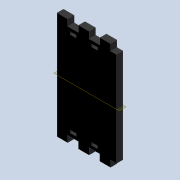
# Autodesk Inventor part: 00_Baseplate_Simmo_side6_v2
Saved by Autodesk Inventor 2022 (Build 260153000, 153)
## iProperties
Created: 2022-08-09
Part Number: 00_Baseplate_Simmo_side6_v2
Material: Generic
Document SubType Name: Modeling
Designer: wanghaoran
Density: 1 g/cm^3
Appearance: Default
Author: wanghaoran
Autodesk Inventor part; units mm, degrees
ref_plane "YZ Plane" through (0, 0, 0) normal (1, 0, 0) x (0, 1, 0)
ref_plane "XZ Plane" through (0, 0, 0) normal (0, 1, 0) x (-1, 0, 0)
ref_plane "XY Plane" through (0, 0, 0) normal (0, 0, 1) x (1, 0, 0)
sketch "Sketch1" plane through (0, 0, 0) normal (0, 0, 1) x (1, 0, 0)
  line L0 (50, 0) -> (55.5309, 0) projected
  line L1 (0, 0) -> (0, 6) projected
  line L2 (0, 0) -> (0, 6) projected
  line L3 (0, 0) -> (0, 6) projected
  line L4 (0, 6) -> (55.5309, 6)
  line L5 (55.5309, 6) -> (55.5309, -94)
  line L6 (55.5309, -94) -> (0, -94)
  line L7 (0, -94) -> (0, 6)
  line L8 (55.5309, 6) -> (55.5309, 0) projected
  line L9 (55.5309, 6) -> (55.5309, 0) projected
  dimension "d16" = 100
  constraints: 8 end point, 2 parallel, 1 horizontal, 1 perpendicular
  measures "d16" distance of L4.end L5.end
extrude "Extrusion1" add sketch "Sketch1" along normal blind 6
sketch "Sketch2" plane through (0, 0, 6) normal (0, 0, 1) x (1, 0, 0)
  line L0 (50, 0) -> (55.5309, 0) projected
  line L1 (50, 6) -> (50, 0) projected
  line L2 (58.2654, -73) -> (58.2654, 6) projected
  line L3 (58.2654, 6) -> (0, 6) projected
  line L4 (30, 6) -> (30, 0) projected
  line L5 (30, 0) -> (40, 0) projected
  line L6 (40, 0) -> (40, 6) projected
  line L7 (50, 0) -> (49.9, 0)
  line L8 (49.9, 0) -> (49.9, 6)
  line L9 (49.9, 6) -> (50, 6)
  line L10 (50, 6) -> (50, 0)
  line L11 (40, 0) -> (40.1, 0)
  line L12 (40.1, 0) -> (40.1, 6)
  line L13 (40.1, 6) -> (40, 6)
  line L14 (40, 6) -> (40, 0)
  line L15 (30, 0) -> (29.9, 0)
  line L16 (29.9, 0) -> (29.9, 6)
  line L17 (29.9, 6) -> (30, 6)
  line L18 (30, 6) -> (30, 0)
  line L19 (10, 6) -> (10, 0) projected
  line L20 (20, 0) -> (20, 6) projected
  line L21 (10, 0) -> (20, 0) projected
  line L22 (20, 0) -> (20.1, 0)
  line L23 (20.1, 0) -> (20.1, 6)
  line L24 (20.1, 6) -> (20, 6)
  line L25 (20, 6) -> (20, 0)
  line L26 (10, 0) -> (9.9, 0)
  line L27 (9.9, 0) -> (9.9, 6)
  line L28 (9.9, 6) -> (10, 6)
  line L29 (10, 6) -> (10, 0)
  line L30 (55.5309, -94) -> (55.5309, 6) projected
  point P0 (40.1, 6)
  point P1 (29.9, 6)
  point P2 (49.9, 6)
  point P3 (49.9, 0.06)
  point P4 (30.1, 0)
  point P5 (39.9, 0)
  point P6 (39.9, 0.03)
  point P7 (30.1, 2.97)
  point P8 (30, 6)
  point P9 (40, 0)
  point P10 (58.2654, 0)
  dimension "d3" = 0.1
  dimension "d4" = 6
  dimension "d5" = 0.1
  dimension "d6" = 6
  dimension "d7" = 0.1
  dimension "d8" = 6
  dimension "d17" = 0.1
  dimension "d18" = 6
  dimension "d19" = 0.1
  dimension "d20" = 6
  constraints: 40 end point, 10 parallel, 5 horizontal, 5 perpendicular, 1 other
  measures "d3" distance of L8.end L9.end
  measures "d4" distance of L7.end L8.end
  measures "d5" distance of L13.end L12.end
  measures "d6" distance of L12.end L11.end
  measures "d7" distance of L16.end L17.end
  measures "d8" distance of L15.end L16.end
  measures "d17" distance of L24.end L23.end
  measures "d18" distance of L23.end L22.end
  measures "d19" distance of L27.end L28.end
  measures "d20" distance of L26.end L27.end
extrude "Extrusion2" cut sketch "Sketch2" against normal through all
ref_plane "Work Plane1" through (0, -44, 0) normal (0, -1, 0) x (1, 0, 0)
mirror "Mirror1" about plane through (0, -44, 0) normal (0, -1, 0) of "Extrusion2"
sketch "Sketch3" plane through (0, 0, 6) normal (0, 0, 1) x (1, 0, 0)
  line L0 (37.75, -5.4) -> (32.25, -5.4)
  line L1 (32.25, -5.4) -> (32.25, -3)
  line L2 (32.25, -3) -> (37.75, -3)
  line L3 (37.75, -3) -> (37.75, -5.4)
  line L4 (40.1, 6) -> (40.1, 0) projected
  line L5 (40.1, 0) -> (29.9, 0) projected
  point P0 (0, 0)
  dimension "d21" = 5.5
  dimension "d22" = 2.4
  dimension "d23" = 2.35
  dimension "d24" = 3
  constraints: 8 end point, 2 parallel, 1 horizontal, 1 perpendicular
  measures "d21" distance of L1.end L2.end
  measures "d22" distance of L0.end L1.end
  measures "d23" distance between parallel lines of L4 L3
  measures "d24" distance between parallel lines of L5 L2
extrude "Extrusion3" cut sketch "Sketch3" against normal through all
pattern_linear "Rectangular Pattern1" count 2 spacing 20 along (-1, 0, 0) of "Extrusion3"
mirror "Mirror2" about plane through (0, -44, 0) normal (0, -1, 0) of "Extrusion3", "Rectangular Pattern1"
body "Solid1"
